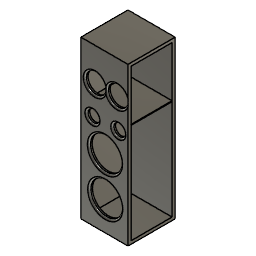
Tower Design (Autodesk Fusion 360 design; units mm, degrees)
part number: 2026-03-23-18-15-23-053
Autodesk Fusion 360 part; units mm, degrees
sketch "Sketch1" plane through (0, 0, 0) normal (0, 0, 1) x (1, 0, 0)
  line L0 (-150, 150) -> (150, 150)
  line L1 (150, 150) -> (150, -150)
  line L2 (150, -150) -> (-150, -150)
  line L3 (-150, -150) -> (-150, 150)
  dimension "d1" = 300
  dimension "d2" = 300
  dimension "d3" = 150
  dimension "d4" = 150
  constraint horizontal L0
  constraint vertical L1
  constraint horizontal L2
  constraint vertical L3
  measures "d1" distance of L0.start L0.end
  measures "d2" distance of L0.start L2.end
  measures "d3" distance of origin L0
  measures "d4" distance of origin L3
extrude "Extrude1" add sketch "Sketch1" along normal blind 1000 makes body 1
shell "Shell1" thickness 20 removed faces 1 at (150, 50, 333.3333) on bodies 1
hole "Hole1" at (5.464, -150, 185.8192) direction (0, 1, 0) diameter 203 depth 100 tip angle 180 bodies 1
hole "Hole2" at (3.4945, -150, 431.7606) direction (0, 1, 0) diameter 203 depth 100 tip angle 180 bodies 1
hole "Hole3" at (-75.7337, -150, 598.4129) direction (0, 1, 0) diameter 76 depth 100 tip angle 180 bodies 1
hole "Hole4" at (88.1867, -150, 603.877) direction (0, 1, 0) diameter 76 depth 100 tip angle 180 bodies 1
hole "Hole5" at (-60.7058, -150, 786.9315) direction (0, 1, 0) diameter 127 depth 100 tip angle 180 bodies 1
hole "Hole6" at (79.9907, -150, 788.2875) direction (0, 1, 0) diameter 127 depth 100 tip angle 180 bodies 1
sketch "Sketch2" plane through (0, 0, 20) normal (0, 0, 1) x (-1, 0, 0)
  line L0 (130, 130) -> (-150, 130)
  line L1 (-150, 130) -> (-150, -130)
  line L2 (-150, -130) -> (130, -130)
  line L3 (130, -130) -> (130, 130)
  line L4 (150, -150) -> (-150, -150)
  line L5 (-150, -150) -> (-150, 150)
  line L6 (-150, 150) -> (150, 150)
  line L7 (150, 150) -> (150, -150)
  constraint horizontal L4
  constraint vertical L5
  constraint horizontal L6
  constraint vertical L7
extrude "Extrude2" add sketch "Sketch2" along normal blind 5 separate body contours L0 L1 L2 L3 L5 makes body 2
move_body "Move1" bodies 2 to x (1, 0, 0) y (0, 1, 0) z (0, 0, 1) at (0, 0, 635)
fillet "Fillet1" radius 10 1 edges at (-37.7432, -150, 846.1343) on bodies 1
fillet "Fillet2" radius 10 1 edges at (102.9533, -150, 847.4903) on bodies 1
fillet "Fillet3" radius 10 4 edges at (-61.9923, -150, 633.8413) (101.9281, -150, 639.3054) (40.1985, -150, 526.3918) (42.168, -150, 280.4504) on bodies 1
